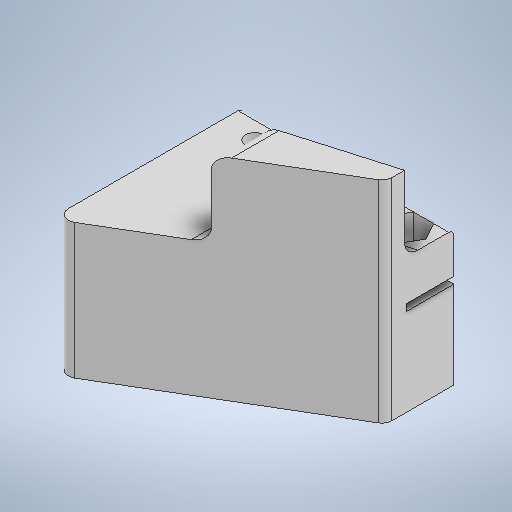
# Autodesk Inventor part: mogo aligner
Saved by Autodesk Inventor 2025.2 (Build 292293000, 293)
## iProperties
Created: 2024-12-10
Part Number: mogo aligner
Material: Generic
Document SubType Name: Modeling
Designer: hmath
Density: 1 g/cm^3
Appearance: Default
Author: hmath
Autodesk Inventor part; units mm, degrees
ref_plane "YZ Plane" through (0, 0, 0) normal (1, 0, 0) x (0, 1, 0)
ref_plane "XZ Plane" through (0, 0, 0) normal (0, 1, 0) x (-1, 0, 0)
ref_plane "XY Plane" through (0, 0, 0) normal (0, 0, 1) x (1, 0, 0)
sketch "Sketch1" plane through (0, 0, 0) normal (0, 0, 1) x (1, 0, 0)
  line L0 (0, 0) -> (52.959, 0)
  line L1 (52.959, 0) -> (52.959, 21.717)
  line L2 (52.959, 21.717) -> (0, 21.717)
  line L3 (0, 21.717) -> (0, 0)
  dimension "d0" = 52.959
  dimension "d1" = 21.717
  constraints: 8 end point, 2 parallel, 1 horizontal, 1 perpendicular
  measures "d0" distance of L1.end L2.end
  measures "d1" distance of L0.end L1.end
extrude "Extrusion1" add sketch "Sketch1" along normal blind 11.9126
sketch "Sketch3" plane through (0, 21.717, 0) normal (0, 1, 0) x (1, 0, 0)
  line L0 (52.959, -11.9126) -> (0, -11.9126) projected
  line L1 (52.959, -11.9126) -> (25.3122, -11.9126)
  line L2 (25.3122, -25.5065) -> (25.3122, -11.9126)
  line L3 (25.3122, -25.5065) -> (25.3122, -33.3756)
  line L4 (52.959, -11.9126) -> (52.959, -16.9926)
  line L5 (52.959, -16.9926) -> (25.3122, -33.3756)
  line L6 (25.3122, -33.3756) -> (25.3122, -34.9664)
  point P0 (0, 0)
  dimension "d20" = 5.08
  dimension "d21" = 21.463
  constraints: 12 end point, 2 vertical, 1 parallel, 1 perpendicular, 1 point on line
  measures "d20" distance of L0.start L4.end
  measures "d21" distance of L3.end L1.end
extrude "Extrusion2" add sketch "Sketch3" against normal up to surface (21.717 mm away)
sketch "Sketch4" plane through (0, 21.717, 0) normal (0, 1, 0) x (1, 0, 0)
  line L0 (52.959, 0) -> (52.959, -16.9926) projected
  line L1 (52.959, 0) -> (52.959, -5.5626)
  line L2 (52.959, -5.5626) -> (46.609, -5.5626)
  circle A0 centre (46.609, -5.5626) radius 2.3241
  line L3 (52.959, 0) -> (0, 0) projected
  circle A1 centre (33.909, -5.5626) radius 2.3241
  circle A2 centre (21.209, -5.5626) radius 2.3241
  circle A3 centre (8.509, -5.5626) radius 2.3241
  point P0 (52.959, -11.0236)
  dimension "d8" = 6.35
  dimension "d9" = 4.6482
  dimension "d12" = 5.5626
  dimension "d15" = 12.7
  constraints: 4 centre point, 4 end point, 1 coincident, 1 horizontal, 1 perpendicular, 1 point on line, 6 other
  measures "d8" distance of L1.end L2.end
  measures "d9" diameter of A0
  measures "d12" distance between parallel lines of L3 L2
  measures "d15" distance of A0.centre A1.centre
extrude "Extrusion3" cut sketch "Sketch4" along normal blind 25.4 and the other way blind 25.4 contours A0
sketch "Sketch7" plane through (0, 21.717, 0) normal (0, 1, 0) x (1, 0, 0)
  line L0 (52.959, 0) -> (52.959, -16.9926) projected
  line L1 (25.3122, -33.3756) -> (52.959, -16.9926) projected
  line L2 (52.959, -16.9926) -> (25.3122, -33.3756)
  line L3 (25.3122, -33.3756) -> (0, -48.3751)
  line L4 (0, 0) -> (0, -11.9126) projected
  line L5 (0, -48.3751) -> (0, -11.9126)
  line L6 (0, -11.9126) -> (25.3122, -11.9126)
  line L7 (25.3122, -11.9126) -> (52.959, -11.9126)
  line L8 (52.959, -11.9126) -> (52.959, -16.9926)
  constraints: 12 end point, 2 collinear, 2 perpendicular, 2 point on line
extrude "Extrusion5" add sketch "Sketch7" along normal blind 11.9126
sketch "Sketch8" plane through (0, 21.717, 0) normal (0, -1, 0) x (1, 0, 0)
  line L0 (0, 48.3751) -> (52.959, 16.9926) projected
  line L1 (0, 11.9126) -> (25.3122, 11.9126) projected
  line L2 (0, 48.3751) -> (0, 11.9126)
  line L3 (25.3122, 11.9126) -> (52.959, 11.9126) projected
  line L4 (0, 11.9126) -> (25.3122, 11.9126)
  line L5 (25.3122, 11.9126) -> (25.3122, 33.3756) projected
  line L6 (25.3122, 11.9126) -> (25.3122, 33.3756)
  line L7 (0, 48.3751) -> (25.3122, 33.3756) projected
  line L8 (25.3122, 33.3756) -> (0, 48.3751)
  point P0 (0, 0)
  constraints: 8 end point, 2 collinear, 1 perpendicular, 1 vertical
extrude "Extrusion6" add sketch "Sketch8" along normal up to surface (21.717 mm away)
sketch "Sketch10" plane through (52.959, 21.717, 11.9126) normal (0, 0, -1) x (-1, 0, 0)
  line L0 (52.959, 0) -> (52.959, 1.6933)
  line L1 (52.959, 0) -> (52.959, 11.9126) projected
  line L2 (52.959, 1.6933) -> (52.959, 11.9126)
  line L3 (0, 11.9126) -> (52.959, 11.9126) projected
  line L4 (52.959, 11.9126) -> (0, 11.9126)
  line L5 (0, 11.9126) -> (0, 1.6933)
  line L6 (0, 1.6933) -> (52.959, 1.6933)
  point P0 (52.959, -21.717)
  dimension "d39" = 1.6933
  constraints: 10 end point, 2 perpendicular, 1 collinear, 1 horizontal, 1 point on line
  measures "d39" distance of L0.start L0.end
extrude "Extrusion9" add sketch "Sketch10" along normal up to surface (11.9126 mm away)
fillet "Fillet6" radius 2.54 2 edges at (52.959, 16.8148, 16.9926) (0, 16.8148, 48.3751)
extrude "Extrusion8" cut sketch "Sketch4" along normal blind 12.7 contours A3
fillet "Fillet7" radius 1.27 1 edges at (26.4795, 33.6296, 0)
sketch "Sketch11" plane through (0, 33.6296, 0) normal (0, 1, 0) x (1, 0, 0)
  arc A0 (10.7824, -5.08) -> (6.2356, -5.08) centre (8.509, -5.5626) ccw projected
  line L0 (8.509, -5.5626) -> (46.609, -5.5626)
  circle A1 centre (46.609, -5.5626) radius 2.3241 projected
  circle A2 centre (46.609, -5.5626) radius 2.3241
  point P0 (0, 0)
  dimension "d46" = 38.1
  constraints: 2 end point, 1 centre point, 1 coincident, 1 horizontal
  measures "d46" distance of L0.start L0.end
extrude "Extrusion10" cut sketch "Sketch11" against normal blind 33.6296
sketch "Sketch12" plane through (0, 0, 0) normal (0, -1, 0) x (1, 0, 0)
  line L0 (52.959, 11.9126) -> (52.959, 0) projected
  line L1 (52.959, 0) -> (52.959, 11.9126)
  line L2 (0, 43.9175) -> (0, 1.27) projected
  line L3 (0, 11.9126) -> (0, 0)
  line L4 (0, 0) -> (52.959, 0)
  line L5 (0, 0) -> (0, 43.9175) projected
  line L6 (0, 11.9126) -> (0, 43.9175)
  arc A0 (52.959, 15.5453) -> (51.7139, 17.7304) centre (50.419, 15.5453) ccw projected
  line L7 (52.959, 11.9126) -> (52.959, 15.5453)
  arc A1 (52.959, 15.5453) -> (51.7139, 17.7304) centre (50.419, 15.5453) ccw
  arc A2 (3.8349, 46.1026) -> (0, 43.9175) centre (2.54, 43.9175) ccw projected
  arc A3 (3.8349, 46.1026) -> (0, 43.9175) centre (2.54, 43.9175) ccw
  line L8 (3.8349, 46.1026) -> (51.7139, 17.7304) projected
  line L9 (3.8349, 46.1026) -> (51.7139, 17.7304)
  point P0 (0, 1.27)
  constraints: 12 end point, 4 collinear, 4 point on circle, 4 tangent, 2 centre point, 1 perpendicular, 1 point on line, 1 vertical
extrude "Extrusion11" add sketch "Sketch12" along normal blind 0.254
sketch "Sketch13" plane through (0, -0.254, 0) normal (0, -1, 0) x (1, 0, 0)
  circle A0 centre (46.609, 5.5626) radius 2.3241 projected
  point P0 (0, 0)
extrude "Extrusion12" cut sketch "Sketch13" against normal blind 33.6296
sketch "Sketch15" plane through (0, 21.717, 0) normal (-1, 0, 0) x (0, 0, 1)
  circle A0 centre (5.9563, 6.2571) radius 2.3241
  point P0 (0, -21.717)
  dimension "d57" = 4.6482
  constraints: 1 centre point
  measures "d57" diameter of A0
extrude "Extrusion14" cut sketch "Sketch15" against normal blind 8.89
sketch "Sketch16" plane through (0, 33.6296, 0) normal (0, 1, 0) x (1, 0, 0)
  circle A0 centre (46.609, -5.5626) radius 2.3241 projected
  circle A1 centre (46.609, -5.5626) radius 4.1275
  line L0 (0, -1.27) -> (52.959, -1.27) projected
  line L1 (49.1448, -1.27) -> (51.5944, -5.6123)
  line L2 (51.5944, -5.6123) -> (49.0586, -9.9049)
  line L3 (49.0586, -9.9049) -> (44.0732, -9.8552)
  line L4 (44.0732, -9.8552) -> (41.6236, -5.5129)
  line L5 (41.6236, -5.5129) -> (44.1594, -1.2203)
  line L6 (44.1594, -1.2203) -> (49.1448, -1.27)
  point P0 (0, 0)
  point P1 (44.13, -1.27)
  dimension "d60" = 8.255
  constraints: 12 end point, 3 coincident, 1 centre point, 1 point on line, 13 other
  measures "d60" diameter of A1
extrude "Extrusion15" cut sketch "Sketch16" against normal blind 6.35 contours A1 | L0 L1 L2 L3 L4 L5
sketch "Sketch17" plane through (0, 33.6296, 0) normal (0, 1, 0) x (1, 0, 0)
  arc A0 (51.7139, -17.7304) -> (52.959, -15.5453) centre (50.419, -15.5453) ccw projected
  line L0 (52.959, 0) -> (52.959, -15.5453) projected
  line L1 (52.959, -15.5453) -> (52.959, -12.3703)
  line L2 (52.959, -12.3703) -> (25.3745, -20.4322)
  line L3 (25.3745, -20.4322) -> (25.3745, -33.3386)
  line L4 (3.8349, -46.1026) -> (51.7139, -17.7304) projected
  line L5 (25.3745, -33.3386) -> (51.7139, -17.7304)
  point P0 (0, 0)
  dimension "d63" = 3.175
  constraints: 8 end point, 2 point on line, 1 collinear, 1 parallel, 1 tangent
  measures "d63" distance of L0.end L1.end
extrude "Extrusion16" add sketch "Sketch17" along normal blind 19.05
fillet "Fillet8" radius 3.175 3 edges at (25.3745, 33.6296, 26.8854) (39.1668, 33.6296, 16.4012) (25.3745, 52.6796, 26.8854)
body "Solid1"
